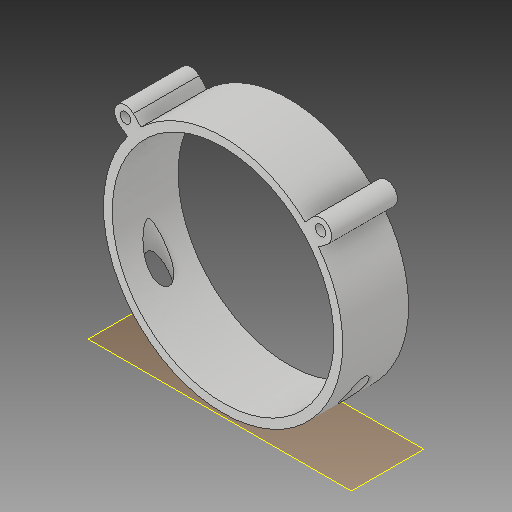
# Autodesk Inventor part: peristalticPumpExtension
Saved by Autodesk Inventor 2017 (Build 210142000, 142)
## iProperties
Created: 2016-11-08
Part Number: peristalticPumpExtension
Material: Generic
Document SubType Name: Modeling
Designer: Camilo
Density: 1 g/cm^3
Appearance: Default
Author: Camilo
Autodesk Inventor part; units mm, degrees
ref_plane "YZ Plane" through (0, 0, 0) normal (1, 0, 0) x (0, 1, 0)
ref_plane "XY Plane" through (0, 0, 0) normal (0, 0, 1) x (1, 0, 0)
sketch "Sketch1" plane through (0, 0, 0) normal (0, 0, 1) x (1, 0, 0)
  line L0 (3.8685, 0) -> (1.9343, -3.3502) construction
  line L1 (1.9343, -3.3502) -> (-1.9342, -3.3502) construction
  line L2 (-1.9342, -3.3502) -> (-3.8685, 0) construction
  line L3 (-3.8685, 0) -> (-1.9342, 3.3502) construction
  line L4 (-1.9342, 3.3502) -> (1.9343, 3.3502) construction
  line L5 (1.9343, 3.3502) -> (3.8685, 0) construction
  circle A0 centre (0, 0) radius 27.135 construction
  circle A1 centre (0, 0) radius 25.235
  circle A2 centre (0, 0) radius 27.235
  point P0 (0, 0)
  dimension "d0" = 0.1
  dimension "d1" = 2
  constraints: 2 centre point, 2 coincident
  measures "d0" radial gap between concentric circles of A0 A2
  measures "d1" radial gap between concentric circles of A2 A1
ref_plane "Work Plane1" through (-27.135, -27.135, -15) normal (0, 0, -1) x (0, 1, 0)
extrude "Extrusion1" add sketch "Sketch1" against normal up to surface (15 mm away)
sketch "Sketch2" plane through (0, 0, 0) normal (0, 0, 1) x (1, 0, 0)
  circle A0 centre (-22.2214, 19.9082) radius 1.2 construction
  circle A1 centre (-22.2214, 19.9082) radius 2.5 construction
  circle A2 centre (22.2214, 19.9082) radius 1.2 construction
  circle A3 centre (22.2214, 19.9082) radius 2.5 construction
  circle A4 centre (0, 0) radius 25.235 construction
  circle A5 centre (0, 0) radius 27.235 construction
  circle A6 centre (22.2214, 19.9082) radius 2.5
  circle A7 centre (-22.2214, 19.9082) radius 2.5
  line L0 (-20.4031, 21.6239) -> (-18.0045, 19.0818)
  line L1 (-23.7277, 17.9129) -> (-20.9383, 15.8071)
  circle A8 centre (0, 0) radius 27.235 construction
  line L2 (23.7277, 17.9129) -> (20.9383, 15.8071)
  line L3 (20.4031, 21.6239) -> (18.0045, 19.0818)
  circle A9 centre (0, 0) radius 26.235
  point P0 (0, 0)
  dimension "d5" = 1
  constraints: 12 point on circle, 8 end point, 4 line through centre, 4 tangent, 3 centre point, 3 coincident, 2 concentric
  measures "d5" radial gap between concentric circles of A5 A9
ref_plane "Work Plane2" through (-27.135, -27.135, -15) normal (0, 0, -1) x (0, 1, 0)
extrude "Extrusion2" add sketch "Sketch2" against normal up to surface (15 mm away) contours A6 | A6 L2 A9 L3 | A9 L1 A7 L0 | A7
sketch "Sketch3" plane through (0, 0, -15) normal (0, 0, -1) x (-1, 0, 0)
  circle A0 centre (-22.2214, 19.9082) radius 1.2 projected
  circle A1 centre (-22.2214, 19.9082) radius 1.2 projected
  circle A2 centre (22.2214, 19.9082) radius 1.2 projected
  point P0 (0, 0)
extrude "Extrusion3" cut sketch "Sketch3" against normal blind 5
sketch "Sketch4" plane through (0, 0, 0) normal (0, 0, 1) x (1, 0, 0)
  circle A0 centre (22.2214, 19.9082) radius 1.2 projected
  circle A1 centre (-22.2214, 19.9082) radius 1.2 projected
  point P0 (0, 0)
extrude "Extrusion4" cut sketch "Sketch4" against normal blind 4
ref_plane "Work Plane3" through (0, -27.235, 0) normal (0, 1, 0) x (-1, 0, 0)
sketch "Sketch5" plane through (0, -27.235, 0) normal (0, 1, 0) x (-1, 0, 0)
  line L0 (-24.7214, 0) -> (-24.7214, -15) construction
  line L1 (24.7214, 0) -> (24.7214, -15) construction
  line L2 (24.7214, -7.5) -> (-24.7214, -7.5) construction
  circle A0 centre (22.2214, -7.5) radius 2.5
  circle A1 centre (-22.2214, -7.5) radius 2.5
  point P0 (0, 0)
  dimension "d12" = 2.5
  dimension "d13" = 2.5
  dimension "d14" = 5
  constraints: 2 centre point, 2 end point, 2 midpoint, 2 point on line, 1 equal radius
  measures "d12" distance from line of L1 A0.centre
  measures "d13" distance from line of L0 A1.centre
  measures "d14" diameter of A1
extrude "Extrusion5" cut sketch "Sketch5" along normal up to surface round surface about axis through (0, 0, 0) along (0, 0, -1) radius 25.235 far side no
body "Solid1"
